Autodesk Inventor part; units mm, degrees
(part 2 of 2)
sketch "Sketch5" plane through (0, 0, 0) normal (0, 0, -1) x (-1, 0, 0)
  arc A0 (-2.4, 16.6775) -> (-3.5193, 18.4731) centre (-4.4, 16.6775) ccw projected
  arc A1 (-3.5193, 28.9932) -> (-3.5193, 18.4731) centre (-0.9394, 23.7332) ccw projected
  arc A2 (-3.5193, 28.9932) -> (-2.4, 30.7889) centre (-4.4, 30.7889) ccw projected
  line L0 (-2.4, 30.7889) -> (-2.4, 61.2014) projected
  arc A3 (-0.4014, 63.2014) -> (-2.4, 61.2014) centre (-0.4, 61.2014) ccw projected
  line L1 (-0.4014, 63.2014) -> (15.0542, 63.2118) projected
  line L2 (15.0542, 63.2118) -> (15, 62.8) projected
  line L3 (15, 62.8) -> (15.1704, 61.5059) projected
  line L4 (15.1704, 61.5059) -> (15.6699, 60.3) projected
  line L5 (15.6699, 60.3) -> (16.4645, 59.2645) projected
  line L6 (16.4645, 59.2645) -> (17.5, 58.4699) projected
  line L7 (17.5, 58.4699) -> (18.7059, 57.9704) projected
  line L8 (18.7059, 57.9704) -> (20, 57.8) projected
  line L9 (20, 57.8) -> (21.2941, 57.9704) projected
  line L10 (21.2941, 57.9704) -> (22.5, 58.4699) projected
  line L11 (22.5, 58.4699) -> (23.5355, 59.2645) projected
  line L12 (23.5355, 59.2645) -> (24.3301, 60.3) projected
  line L13 (24.3301, 60.3) -> (24.8296, 61.5059) projected
  line L14 (24.8296, 61.5059) -> (25, 62.8) projected
  line L15 (25, 62.8) -> (24.9458, 63.212) projected
  line L16 (24.9458, 63.212) -> (130.4002, 63.2002) projected
  arc A4 (132.4, 61.2002) -> (130.4002, 63.2002) centre (130.4, 61.2002) ccw projected
  line L17 (132.4, 61.2002) -> (132.4, 57.5029) projected
  line L18 (132.4, 57.5029) -> (131.5, 57.1301) projected
  line L19 (131.5, 57.1301) -> (130.4645, 56.3355) projected
  line L20 (130.4645, 56.3355) -> (129.6699, 55.3) projected
  line L21 (129.6699, 55.3) -> (129.1704, 54.0941) projected
  line L22 (129.1704, 54.0941) -> (129, 52.8) projected
  line L23 (129, 52.8) -> (129.1704, 51.5059) projected
  line L24 (129.1704, 51.5059) -> (129.6699, 50.3) projected
  line L25 (129.6699, 50.3) -> (130.4645, 49.2645) projected
  line L26 (130.4645, 49.2645) -> (131.5, 48.4699) projected
  line L27 (131.5, 48.4699) -> (132.4, 48.0971) projected
  line L28 (132.4, 48.0971) -> (132.4, -5.0172) projected
  arc A5 (131.3636, -6.7698) -> (132.4, -5.0172) centre (130.4, -5.0172) ccw projected
  line L29 (131.3636, -6.7698) -> (128.4686, -8.3615) projected
  arc A6 (127.505, -8.6089) -> (128.4686, -8.3615) centre (127.505, -6.6089) ccw projected
  line L30 (127.505, -8.6089) -> (2.6647, -8.6089) projected
  arc A7 (1.7321, -8.3782) -> (2.6647, -8.6089) centre (2.6647, -6.6089) ccw projected
  line L31 (1.7321, -8.3782) -> (-1.3326, -6.7626) projected
  arc A8 (-2.4, -4.9934) -> (-1.3326, -6.7626) centre (-0.4, -4.9934) ccw projected
  line L32 (-2.4, -4.9934) -> (-2.4, 16.6775) projected
  line L33 (142.6617, 57.45) -> (142.392, 58.1012) projected
  line L34 (142.392, 58.1012) -> (142.3, 58.8) projected
  line L35 (142.3, 58.8) -> (142.392, 59.4988) projected
  line L36 (142.392, 59.4988) -> (142.6617, 60.15) projected
  line L37 (142.6617, 60.15) -> (143.0908, 60.7092) projected
  line L38 (143.0908, 60.7092) -> (143.65, 61.1383) projected
  line L39 (143.65, 61.1383) -> (144.3012, 61.408) projected
  line L40 (144.3012, 61.408) -> (145, 61.5) projected
  line L41 (145, 61.5) -> (145.6988, 61.408) projected
  line L42 (145.6988, 61.408) -> (146.35, 61.1383) projected
  line L43 (146.35, 61.1383) -> (146.9092, 60.7092) projected
  line L44 (146.9092, 60.7092) -> (147.3383, 60.15) projected
  line L45 (147.3383, 60.15) -> (147.608, 59.4988) projected
  line L46 (147.608, 59.4988) -> (147.7, 58.8) projected
  line L47 (147.7, 58.8) -> (147.608, 58.1012) projected
  line L48 (147.608, 58.1012) -> (147.3383, 57.45) projected
  line L49 (147.3383, 57.45) -> (146.9092, 56.8908) projected
  line L50 (146.9092, 56.8908) -> (146.35, 56.4617) projected
  line L51 (146.35, 56.4617) -> (145.6988, 56.192) projected
  line L52 (145.6988, 56.192) -> (145, 56.1) projected
  line L53 (145, 56.1) -> (144.3012, 56.192) projected
  line L54 (144.3012, 56.192) -> (143.65, 56.4617) projected
  line L55 (143.65, 56.4617) -> (143.0908, 56.8908) projected
  line L56 (143.0908, 56.8908) -> (142.6617, 57.45) projected
  line L57 (-13.0908, -9.2908) -> (-12.6617, -9.85) projected
  line L58 (-12.6617, -9.85) -> (-12.392, -10.5012) projected
  line L59 (-12.392, -10.5012) -> (-12.3, -11.2) projected
  line L60 (-12.3, -11.2) -> (-12.392, -11.8988) projected
  line L61 (-12.392, -11.8988) -> (-12.6617, -12.55) projected
  line L62 (-12.6617, -12.55) -> (-13.0908, -13.1092) projected
  line L63 (-13.0908, -13.1092) -> (-13.65, -13.5383) projected
  line L64 (-13.65, -13.5383) -> (-14.3012, -13.808) projected
  line L65 (-14.3012, -13.808) -> (-15, -13.9) projected
  line L66 (-15, -13.9) -> (-15.6988, -13.808) projected
  line L67 (-15.6988, -13.808) -> (-16.35, -13.5383) projected
  line L68 (-16.35, -13.5383) -> (-16.9092, -13.1092) projected
  line L69 (-16.9092, -13.1092) -> (-17.3383, -12.55) projected
  line L70 (-17.3383, -12.55) -> (-17.608, -11.8988) projected
  line L71 (-17.608, -11.8988) -> (-17.7, -11.2) projected
  line L72 (-17.7, -11.2) -> (-17.608, -10.5012) projected
  line L73 (-17.608, -10.5012) -> (-17.3383, -9.85) projected
  line L74 (-17.3383, -9.85) -> (-16.9092, -9.2908) projected
  line L75 (-16.9092, -9.2908) -> (-16.35, -8.8617) projected
  line L76 (-16.35, -8.8617) -> (-15.6988, -8.592) projected
  line L77 (-15.6988, -8.592) -> (-15, -8.5) projected
  line L78 (-15, -8.5) -> (-14.3012, -8.592) projected
  line L79 (-14.3012, -8.592) -> (-13.65, -8.8617) projected
  line L80 (-13.65, -8.8617) -> (-13.0908, -9.2908) projected
  line L81 (142.6617, -12.55) -> (142.392, -11.8988) projected
  line L82 (142.392, -11.8988) -> (142.3, -11.2) projected
  line L83 (142.3, -11.2) -> (142.392, -10.5012) projected
  line L84 (142.392, -10.5012) -> (142.6617, -9.85) projected
  line L85 (142.6617, -9.85) -> (143.0908, -9.2908) projected
  line L86 (143.0908, -9.2908) -> (143.65, -8.8617) projected
  line L87 (143.65, -8.8617) -> (144.3012, -8.592) projected
  line L88 (144.3012, -8.592) -> (145, -8.5) projected
  line L89 (145, -8.5) -> (145.6988, -8.592) projected
  line L90 (145.6988, -8.592) -> (146.35, -8.8617) projected
  line L91 (146.35, -8.8617) -> (146.9092, -9.2908) projected
  line L92 (146.9092, -9.2908) -> (147.3383, -9.85) projected
  line L93 (147.3383, -9.85) -> (147.608, -10.5012) projected
  line L94 (147.608, -10.5012) -> (147.7, -11.2) projected
  line L95 (147.7, -11.2) -> (147.608, -11.8988) projected
  line L96 (147.608, -11.8988) -> (147.3383, -12.55) projected
  line L97 (147.3383, -12.55) -> (146.9092, -13.1092) projected
  line L98 (146.9092, -13.1092) -> (146.35, -13.5383) projected
  line L99 (146.35, -13.5383) -> (145.6988, -13.808) projected
  line L100 (145.6988, -13.808) -> (145, -13.9) projected
  line L101 (145, -13.9) -> (144.3012, -13.808) projected
  line L102 (144.3012, -13.808) -> (143.65, -13.5383) projected
  line L103 (143.65, -13.5383) -> (143.0908, -13.1092) projected
  line L104 (143.0908, -13.1092) -> (142.6617, -12.55) projected
  line L105 (143.3271, 8.2886) -> (142.7, 8.5483) projected
  line L106 (142.7, 8.5483) -> (142.1615, 8.9615) projected
  line L107 (142.1615, 8.9615) -> (141.7483, 9.5) projected
  line L108 (141.7483, 9.5) -> (141.4886, 10.1271) projected
  line L109 (141.4886, 10.1271) -> (141.4, 10.8) projected
  line L110 (141.4, 10.8) -> (141.4886, 11.4729) projected
  line L111 (141.4886, 11.4729) -> (141.7483, 12.1) projected
  line L112 (141.7483, 12.1) -> (142.1615, 12.6385) projected
  line L113 (142.1615, 12.6385) -> (142.7, 13.0517) projected
  line L114 (142.7, 13.0517) -> (143.3271, 13.3114) projected
  line L115 (143.3271, 13.3114) -> (144, 13.4) projected
  line L116 (144, 13.4) -> (144.6729, 13.3114) projected
  line L117 (144.6729, 13.3114) -> (145.3, 13.0517) projected
  line L118 (145.3, 13.0517) -> (145.8385, 12.6385) projected
  line L119 (145.8385, 12.6385) -> (146.2517, 12.1) projected
  line L120 (146.2517, 12.1) -> (146.5114, 11.4729) projected
  line L121 (146.5114, 11.4729) -> (146.6, 10.8) projected
  line L122 (146.6, 10.8) -> (146.5114, 10.1271) projected
  line L123 (146.5114, 10.1271) -> (146.2517, 9.5) projected
  line L124 (146.2517, 9.5) -> (145.8385, 8.9615) projected
  line L125 (145.8385, 8.9615) -> (145.3, 8.5483) projected
  line L126 (145.3, 8.5483) -> (144.6729, 8.2886) projected
  line L127 (144.6729, 8.2886) -> (144, 8.2) projected
  line L128 (144, 8.2) -> (143.3271, 8.2886) projected
  line L129 (21.8385, 78.9615) -> (21.3, 78.5483) projected
  line L130 (21.3, 78.5483) -> (20.6729, 78.2886) projected
  line L131 (20.6729, 78.2886) -> (20, 78.2) projected
  line L132 (20, 78.2) -> (19.3271, 78.2886) projected
  line L133 (19.3271, 78.2886) -> (18.7, 78.5483) projected
  line L134 (18.7, 78.5483) -> (18.1615, 78.9615) projected
  line L135 (18.1615, 78.9615) -> (17.7483, 79.5) projected
  line L136 (17.7483, 79.5) -> (17.4886, 80.1271) projected
  line L137 (17.4886, 80.1271) -> (17.4, 80.8) projected
  line L138 (17.4, 80.8) -> (17.4886, 81.4729) projected
  line L139 (17.4886, 81.4729) -> (17.7483, 82.1) projected
  line L140 (17.7483, 82.1) -> (18.1615, 82.6385) projected
  line L141 (18.1615, 82.6385) -> (18.7, 83.0517) projected
  line L142 (18.7, 83.0517) -> (19.3271, 83.3114) projected
  line L143 (19.3271, 83.3114) -> (20, 83.4) projected
  line L144 (20, 83.4) -> (20.6729, 83.3114) projected
  line L145 (20.6729, 83.3114) -> (21.3, 83.0517) projected
  line L146 (21.3, 83.0517) -> (21.8385, 82.6385) projected
  line L147 (21.8385, 82.6385) -> (22.2517, 82.1) projected
  line L148 (22.2517, 82.1) -> (22.5114, 81.4729) projected
  line L149 (22.5114, 81.4729) -> (22.6, 80.8) projected
  line L150 (22.6, 80.8) -> (22.5114, 80.1271) projected
  line L151 (22.5114, 80.1271) -> (22.2517, 79.5) projected
  line L152 (22.2517, 79.5) -> (21.8385, 78.9615) projected
  line L153 (110.6729, 78.2886) -> (110, 78.2) projected
  line L154 (110, 78.2) -> (109.3271, 78.2886) projected
  line L155 (109.3271, 78.2886) -> (108.7, 78.5483) projected
  line L156 (108.7, 78.5483) -> (108.1615, 78.9615) projected
  line L157 (108.1615, 78.9615) -> (107.7483, 79.5) projected
  line L158 (107.7483, 79.5) -> (107.4886, 80.1271) projected
  line L159 (107.4886, 80.1271) -> (107.4, 80.8) projected
  line L160 (107.4, 80.8) -> (107.4886, 81.4729) projected
  line L161 (107.4886, 81.4729) -> (107.7483, 82.1) projected
  line L162 (107.7483, 82.1) -> (108.1615, 82.6385) projected
  line L163 (108.1615, 82.6385) -> (108.7, 83.0517) projected
  line L164 (108.7, 83.0517) -> (109.3271, 83.3114) projected
  line L165 (109.3271, 83.3114) -> (110, 83.4) projected
  line L166 (110, 83.4) -> (110.6729, 83.3114) projected
  line L167 (110.6729, 83.3114) -> (111.3, 83.0517) projected
  line L168 (111.3, 83.0517) -> (111.8385, 82.6385) projected
  line L169 (111.8385, 82.6385) -> (112.2517, 82.1) projected
  line L170 (112.2517, 82.1) -> (112.5114, 81.4729) projected
  line L171 (112.5114, 81.4729) -> (112.6, 80.8) projected
  line L172 (112.6, 80.8) -> (112.5114, 80.1271) projected
  line L173 (112.5114, 80.1271) -> (112.2517, 79.5) projected
  line L174 (112.2517, 79.5) -> (111.8385, 78.9615) projected
  line L175 (111.8385, 78.9615) -> (111.3, 78.5483) projected
  line L176 (111.3, 78.5483) -> (110.6729, 78.2886) projected
  line L177 (-12.7, 8.5483) -> (-13.3271, 8.2886) projected
  line L178 (-13.3271, 8.2886) -> (-14, 8.2) projected
  line L179 (-14, 8.2) -> (-14.6729, 8.2886) projected
  line L180 (-14.6729, 8.2886) -> (-15.3, 8.5483) projected
  line L181 (-15.3, 8.5483) -> (-15.8385, 8.9615) projected
  line L182 (-15.8385, 8.9615) -> (-16.2517, 9.5) projected
  line L183 (-16.2517, 9.5) -> (-16.5114, 10.1271) projected
  line L184 (-16.5114, 10.1271) -> (-16.6, 10.8) projected
  line L185 (-16.6, 10.8) -> (-16.5114, 11.4729) projected
  line L186 (-16.5114, 11.4729) -> (-16.2517, 12.1) projected
  line L187 (-16.2517, 12.1) -> (-15.8385, 12.6385) projected
  line L188 (-15.8385, 12.6385) -> (-15.3, 13.0517) projected
  line L189 (-15.3, 13.0517) -> (-14.6729, 13.3114) projected
  line L190 (-14.6729, 13.3114) -> (-14, 13.4) projected
  line L191 (-14, 13.4) -> (-13.3271, 13.3114) projected
  line L192 (-13.3271, 13.3114) -> (-12.7, 13.0517) projected
  line L193 (-12.7, 13.0517) -> (-12.1615, 12.6385) projected
  line L194 (-12.1615, 12.6385) -> (-11.7483, 12.1) projected
  line L195 (-11.7483, 12.1) -> (-11.4886, 11.4729) projected
  line L196 (-11.4886, 11.4729) -> (-11.4, 10.8) projected
  line L197 (-11.4, 10.8) -> (-11.4886, 10.1271) projected
  line L198 (-11.4886, 10.1271) -> (-11.7483, 9.5) projected
  line L199 (-11.7483, 9.5) -> (-12.1615, 8.9615) projected
  line L200 (-12.1615, 8.9615) -> (-12.7, 8.5483) projected
  line L201 (147.8159, -4.2) -> (147.8159, -7.2) projected
  line L202 (147.8159, -7.2) -> (142.8159, -7.2) projected
  line L203 (142.8159, -7.2) -> (142.8159, -4.2) projected
  line L204 (142.8159, -4.2) -> (147.8159, -4.2) projected
  line L205 (133.2, 51.4144) -> (132.8686, 51.6686) projected
  line L206 (132.8686, 51.6686) -> (132.6144, 52) projected
  line L207 (132.6144, 52) -> (132.4545, 52.3859) projected
  line L208 (132.4545, 52.3859) -> (132.4, 52.8) projected
  line L209 (132.4, 52.8) -> (132.4545, 53.2141) projected
  line L210 (132.4545, 53.2141) -> (132.6144, 53.6) projected
  line L211 (132.6144, 53.6) -> (132.8686, 53.9314) projected
  line L212 (132.8686, 53.9314) -> (133.2, 54.1856) projected
  line L213 (133.2, 54.1856) -> (133.5859, 54.3455) projected
  line L214 (133.5859, 54.3455) -> (134, 54.4) projected
  line L215 (134, 54.4) -> (134.4141, 54.3455) projected
  line L216 (134.4141, 54.3455) -> (134.8, 54.1856) projected
  line L217 (134.8, 54.1856) -> (135.1314, 53.9314) projected
  line L218 (135.1314, 53.9314) -> (135.3856, 53.6) projected
  line L219 (135.3856, 53.6) -> (135.5455, 53.2141) projected
  line L220 (135.5455, 53.2141) -> (135.6, 52.8) projected
  line L221 (135.6, 52.8) -> (135.5455, 52.3859) projected
  line L222 (135.5455, 52.3859) -> (135.3856, 52) projected
  line L223 (135.3856, 52) -> (135.1314, 51.6686) projected
  line L224 (135.1314, 51.6686) -> (134.8, 51.4144) projected
  line L225 (134.8, 51.4144) -> (134.4141, 51.2545) projected
  line L226 (134.4141, 51.2545) -> (134, 51.2) projected
  line L227 (134, 51.2) -> (133.5859, 51.2545) projected
  line L228 (133.5859, 51.2545) -> (133.2, 51.4144) projected
  line L229 (20, 61.2) -> (19.5859, 61.2545) projected
  line L230 (19.5859, 61.2545) -> (19.2, 61.4144) projected
  line L231 (19.2, 61.4144) -> (18.8686, 61.6686) projected
  line L232 (18.8686, 61.6686) -> (18.6144, 62) projected
  line L233 (18.6144, 62) -> (18.4545, 62.3859) projected
  line L234 (18.4545, 62.3859) -> (18.4, 62.8) projected
  line L235 (18.4, 62.8) -> (18.4545, 63.2141) projected
  line L236 (18.4545, 63.2141) -> (18.6144, 63.6) projected
  line L237 (18.6144, 63.6) -> (18.8686, 63.9314) projected
  line L238 (18.8686, 63.9314) -> (19.2, 64.1856) projected
  line L239 (19.2, 64.1856) -> (19.5859, 64.3455) projected
  line L240 (19.5859, 64.3455) -> (20, 64.4) projected
  line L241 (20, 64.4) -> (20.4141, 64.3455) projected
  line L242 (20.4141, 64.3455) -> (20.8, 64.1856) projected
  line L243 (20.8, 64.1856) -> (21.1314, 63.9314) projected
  line L244 (21.1314, 63.9314) -> (21.3856, 63.6) projected
  line L245 (21.3856, 63.6) -> (21.5455, 63.2141) projected
  line L246 (21.5455, 63.2141) -> (21.6, 62.8) projected
  line L247 (21.6, 62.8) -> (21.5455, 62.3859) projected
  line L248 (21.5455, 62.3859) -> (21.3856, 62) projected
  line L249 (21.3856, 62) -> (21.1314, 61.6686) projected
  line L250 (21.1314, 61.6686) -> (20.8, 61.4144) projected
  line L251 (20.8, 61.4144) -> (20.4141, 61.2545) projected
  line L252 (20.4141, 61.2545) -> (20, 61.2) projected
  line L253 (-5.1314, -12.3314) -> (-5.3856, -12) projected
  line L254 (-5.3856, -12) -> (-5.5455, -11.6141) projected
  line L255 (-5.5455, -11.6141) -> (-5.6, -11.2) projected
  line L256 (-5.6, -11.2) -> (-5.5455, -10.7859) projected
  line L257 (-5.5455, -10.7859) -> (-5.3856, -10.4) projected
  line L258 (-5.3856, -10.4) -> (-5.1314, -10.0686) projected
  line L259 (-5.1314, -10.0686) -> (-4.8, -9.8144) projected
  line L260 (-4.8, -9.8144) -> (-4.4141, -9.6545) projected
  line L261 (-4.4141, -9.6545) -> (-4, -9.6) projected
  line L262 (-4, -9.6) -> (-3.5859, -9.6545) projected
  line L263 (-3.5859, -9.6545) -> (-3.2, -9.8144) projected
  line L264 (-3.2, -9.8144) -> (-2.8686, -10.0686) projected
  line L265 (-2.8686, -10.0686) -> (-2.6144, -10.4) projected
  line L266 (-2.6144, -10.4) -> (-2.4545, -10.7859) projected
  line L267 (-2.4545, -10.7859) -> (-2.4, -11.2) projected
  line L268 (-2.4, -11.2) -> (-2.4545, -11.6141) projected
  line L269 (-2.4545, -11.6141) -> (-2.6144, -12) projected
  line L270 (-2.6144, -12) -> (-2.8686, -12.3314) projected
  line L271 (-2.8686, -12.3314) -> (-3.2, -12.5856) projected
  line L272 (-3.2, -12.5856) -> (-3.5859, -12.7455) projected
  line L273 (-3.5859, -12.7455) -> (-4, -12.8) projected
  line L274 (-4, -12.8) -> (-4.4141, -12.7455) projected
  line L275 (-4.4141, -12.7455) -> (-4.8, -12.5856) projected
  line L276 (-4.8, -12.5856) -> (-5.1314, -12.3314) projected
  line L277 (135.3856, -10.4) -> (135.5455, -10.7859) projected
  line L278 (135.5455, -10.7859) -> (135.6, -11.2) projected
  line L279 (135.6, -11.2) -> (135.5455, -11.6141) projected
  line L280 (135.5455, -11.6141) -> (135.3856, -12) projected
  line L281 (135.3856, -12) -> (135.1314, -12.3314) projected
  line L282 (135.1314, -12.3314) -> (134.8, -12.5856) projected
  line L283 (134.8, -12.5856) -> (134.4141, -12.7455) projected
  line L284 (134.4141, -12.7455) -> (134, -12.8) projected
  line L285 (134, -12.8) -> (133.5859, -12.7455) projected
  line L286 (133.5859, -12.7455) -> (133.2, -12.5856) projected
  line L287 (133.2, -12.5856) -> (132.8686, -12.3314) projected
  line L288 (132.8686, -12.3314) -> (132.6144, -12) projected
  line L289 (132.6144, -12) -> (132.4545, -11.6141) projected
  line L290 (132.4545, -11.6141) -> (132.4, -11.2) projected
  line L291 (132.4, -11.2) -> (132.4545, -10.7859) projected
  line L292 (132.4545, -10.7859) -> (132.6144, -10.4) projected
  line L293 (132.6144, -10.4) -> (132.8686, -10.0686) projected
  line L294 (132.8686, -10.0686) -> (133.2, -9.8144) projected
  line L295 (133.2, -9.8144) -> (133.5859, -9.6545) projected
  line L296 (133.5859, -9.6545) -> (134, -9.6) projected
  line L297 (134, -9.6) -> (134.4141, -9.6545) projected
  line L298 (134.4141, -9.6545) -> (134.8, -9.8144) projected
  line L299 (134.8, -9.8144) -> (135.1314, -10.0686) projected
  line L300 (135.1314, -10.0686) -> (135.3856, -10.4) projected
  line L301 (-18, 19.2664) -> (-13, 19.2664) projected
  arc A9 (-18, 19.2664) -> (-20, 17.2664) centre (-18, 17.2664) ccw projected
  line L302 (-20, -15.2) -> (-20, 17.2664) projected
  line L303 (-19.9319, -15.7176) -> (-20, -15.2) projected
  line L304 (-19.8478, -15.9654) -> (-19.9319, -15.7176) projected
  line L305 (-19.7321, -16.2) -> (-19.8478, -15.9654) projected
  line L306 (-19.5867, -16.4175) -> (-19.7321, -16.2) projected
  line L307 (-19.4142, -16.6142) -> (-19.5867, -16.4175) projected
  line L308 (-19.2175, -16.7867) -> (-19.4142, -16.6142) projected
  line L309 (-19, -16.9321) -> (-19.2175, -16.7867) projected
  line L310 (-18.7654, -17.0478) -> (-19, -16.9321) projected
  line L311 (-18.5176, -17.1319) -> (-18.7654, -17.0478) projected
  line L312 (-18, -17.2) -> (-18.5176, -17.1319) projected
  line L313 (148, -17.2) -> (-18, -17.2) projected
  line L314 (148.5176, -17.1319) -> (148, -17.2) projected
  line L315 (148.7654, -17.0478) -> (148.5176, -17.1319) projected
  line L316 (149, -16.9321) -> (148.7654, -17.0478) projected
  line L317 (149.2175, -16.7867) -> (149, -16.9321) projected
  line L318 (149.4142, -16.6142) -> (149.2175, -16.7867) projected
  line L319 (149.5867, -16.4175) -> (149.4142, -16.6142) projected
  line L320 (149.7321, -16.2) -> (149.5867, -16.4175) projected
  line L321 (149.8478, -15.9654) -> (149.7321, -16.2) projected
  line L322 (149.9319, -15.7176) -> (149.8478, -15.9654) projected
  line L323 (150, -15.2) -> (149.9319, -15.7176) projected
  line L324 (150, 86.8) -> (150, -15.2) projected
  line L325 (149.9319, 87.3176) -> (150, 86.8) projected
  line L326 (149.8478, 87.5654) -> (149.9319, 87.3176) projected
  line L327 (149.7321, 87.8) -> (149.8478, 87.5654) projected
  line L328 (149.5867, 88.0175) -> (149.7321, 87.8) projected
  line L329 (149.4142, 88.2142) -> (149.5867, 88.0175) projected
  line L330 (149.2175, 88.3867) -> (149.4142, 88.2142) projected
  line L331 (149, 88.5321) -> (149.2175, 88.3867) projected
  line L332 (148.7654, 88.6478) -> (149, 88.5321) projected
  line L333 (148.5176, 88.7319) -> (148.7654, 88.6478) projected
  line L334 (148, 88.8) -> (148.5176, 88.7319) projected
  line L335 (-9, 88.8) -> (148, 88.8) projected
  arc A10 (-9, 88.8) -> (-11, 86.8) centre (-9, 86.8) ccw projected
  line L336 (-11, 21.2664) -> (-11, 86.8) projected
  arc A11 (-13, 19.2664) -> (-11, 21.2664) centre (-13, 21.2664) ccw projected
  circle A12 centre (134, -11.2) radius 1.5863
  circle A13 centre (134, 52.8) radius 1.5863
  circle A14 centre (20, 62.8) radius 1.5863
  circle A15 centre (-4, -11.2) radius 1.5863
  point P0 (0, 0)
  constraints: 12 tangent, 4 centre point
hole "Hole1" at (-134, 52.8, 0) at (-134, -11.2, 0) at (-20, 62.8, 0) at (4, -11.2, 0) direction (0, 0, 1) diameter 3.3 end through all
sketch "Sketch6" plane through (0, 0, 0) normal (0, 0, -1) x (-1, 0, 0)
  circle A0 centre (20, 62.8) radius 1.65 projected
  circle A1 centre (134, 52.8) radius 1.65 projected
  circle A2 centre (134, -11.2) radius 1.65 projected
  circle A3 centre (-4, -11.2) radius 1.65 projected
  arc A4 (-2.4, 16.6775) -> (-3.5193, 18.4731) centre (-4.4, 16.6775) ccw projected
  arc A5 (-3.5193, 28.9932) -> (-3.5193, 18.4731) centre (-0.9394, 23.7332) ccw projected
  arc A6 (-3.5193, 28.9932) -> (-2.4, 30.7889) centre (-4.4, 30.7889) ccw projected
  line L0 (-2.4, 30.7889) -> (-2.4, 61.2014) projected
  arc A7 (-0.4014, 63.2014) -> (-2.4, 61.2014) centre (-0.4, 61.2014) ccw projected
  line L1 (-0.4014, 63.2014) -> (15.0542, 63.2118) projected
  line L2 (15.0542, 63.2118) -> (15, 62.8) projected
  line L3 (15, 62.8) -> (15.1704, 61.5059) projected
  line L4 (15.1704, 61.5059) -> (15.6699, 60.3) projected
  line L5 (15.6699, 60.3) -> (16.4645, 59.2645) projected
  line L6 (16.4645, 59.2645) -> (17.5, 58.4699) projected
  line L7 (17.5, 58.4699) -> (18.7059, 57.9704) projected
  line L8 (18.7059, 57.9704) -> (20, 57.8) projected
  line L9 (20, 57.8) -> (21.2941, 57.9704) projected
  line L10 (21.2941, 57.9704) -> (22.5, 58.4699) projected
  line L11 (22.5, 58.4699) -> (23.5355, 59.2645) projected
  line L12 (23.5355, 59.2645) -> (24.3301, 60.3) projected
  line L13 (24.3301, 60.3) -> (24.8296, 61.5059) projected
  line L14 (24.8296, 61.5059) -> (25, 62.8) projected
  line L15 (25, 62.8) -> (24.9458, 63.212) projected
  line L16 (24.9458, 63.212) -> (130.4002, 63.2002) projected
  arc A8 (132.4, 61.2002) -> (130.4002, 63.2002) centre (130.4, 61.2002) ccw projected
  line L17 (132.4, 61.2002) -> (132.4, 57.5029) projected
  line L18 (132.4, 57.5029) -> (131.5, 57.1301) projected
  line L19 (131.5, 57.1301) -> (130.4645, 56.3355) projected
  line L20 (130.4645, 56.3355) -> (129.6699, 55.3) projected
  line L21 (129.6699, 55.3) -> (129.1704, 54.0941) projected
  line L22 (129.1704, 54.0941) -> (129, 52.8) projected
  line L23 (129, 52.8) -> (129.1704, 51.5059) projected
  line L24 (129.1704, 51.5059) -> (129.6699, 50.3) projected
  line L25 (129.6699, 50.3) -> (130.4645, 49.2645) projected
  line L26 (130.4645, 49.2645) -> (131.5, 48.4699) projected
  line L27 (131.5, 48.4699) -> (132.4, 48.0971) projected
  line L28 (132.4, 48.0971) -> (132.4, -5.0172) projected
  arc A9 (131.3636, -6.7698) -> (132.4, -5.0172) centre (130.4, -5.0172) ccw projected
  line L29 (131.3636, -6.7698) -> (128.4686, -8.3615) projected
  arc A10 (127.505, -8.6089) -> (128.4686, -8.3615) centre (127.505, -6.6089) ccw projected
  line L30 (127.505, -8.6089) -> (2.6647, -8.6089) projected
  arc A11 (1.7321, -8.3782) -> (2.6647, -8.6089) centre (2.6647, -6.6089) ccw projected
  line L31 (1.7321, -8.3782) -> (-1.3326, -6.7626) projected
  arc A12 (-2.4, -4.9934) -> (-1.3326, -6.7626) centre (-0.4, -4.9934) ccw projected
  line L32 (-2.4, -4.9934) -> (-2.4, 16.6775) projected
  line L33 (142.6617, 57.45) -> (142.392, 58.1012) projected
  line L34 (142.392, 58.1012) -> (142.3, 58.8) projected
  line L35 (142.3, 58.8) -> (142.392, 59.4988) projected
  line L36 (142.392, 59.4988) -> (142.6617, 60.15) projected
  line L37 (142.6617, 60.15) -> (143.0908, 60.7092) projected
  line L38 (143.0908, 60.7092) -> (143.65, 61.1383) projected
  line L39 (143.65, 61.1383) -> (144.3012, 61.408) projected
  line L40 (144.3012, 61.408) -> (145, 61.5) projected
  line L41 (145, 61.5) -> (145.6988, 61.408) projected
  line L42 (145.6988, 61.408) -> (146.35, 61.1383) projected
  line L43 (146.35, 61.1383) -> (146.9092, 60.7092) projected
  line L44 (146.9092, 60.7092) -> (147.3383, 60.15) projected
  line L45 (147.3383, 60.15) -> (147.608, 59.4988) projected
  line L46 (147.608, 59.4988) -> (147.7, 58.8) projected
  line L47 (147.7, 58.8) -> (147.608, 58.1012) projected
  line L48 (147.608, 58.1012) -> (147.3383, 57.45) projected
  line L49 (147.3383, 57.45) -> (146.9092, 56.8908) projected
  line L50 (146.9092, 56.8908) -> (146.35, 56.4617) projected
  line L51 (146.35, 56.4617) -> (145.6988, 56.192) projected
  line L52 (145.6988, 56.192) -> (145, 56.1) projected
  line L53 (145, 56.1) -> (144.3012, 56.192) projected
  line L54 (144.3012, 56.192) -> (143.65, 56.4617) projected
  line L55 (143.65, 56.4617) -> (143.0908, 56.8908) projected
  line L56 (143.0908, 56.8908) -> (142.6617, 57.45) projected
  line L57 (-13.0908, -9.2908) -> (-12.6617, -9.85) projected
  line L58 (-12.6617, -9.85) -> (-12.392, -10.5012) projected
  line L59 (-12.392, -10.5012) -> (-12.3, -11.2) projected
  line L60 (-12.3, -11.2) -> (-12.392, -11.8988) projected
  line L61 (-12.392, -11.8988) -> (-12.6617, -12.55) projected
  line L62 (-12.6617, -12.55) -> (-13.0908, -13.1092) projected
  line L63 (-13.0908, -13.1092) -> (-13.65, -13.5383) projected
  line L64 (-13.65, -13.5383) -> (-14.3012, -13.808) projected
  line L65 (-14.3012, -13.808) -> (-15, -13.9) projected
  line L66 (-15, -13.9) -> (-15.6988, -13.808) projected
  line L67 (-15.6988, -13.808) -> (-16.35, -13.5383) projected
  line L68 (-16.35, -13.5383) -> (-16.9092, -13.1092) projected
  line L69 (-16.9092, -13.1092) -> (-17.3383, -12.55) projected
  line L70 (-17.3383, -12.55) -> (-17.608, -11.8988) projected
  line L71 (-17.608, -11.8988) -> (-17.7, -11.2) projected
  line L72 (-17.7, -11.2) -> (-17.608, -10.5012) projected
  line L73 (-17.608, -10.5012) -> (-17.3383, -9.85) projected
  line L74 (-17.3383, -9.85) -> (-16.9092, -9.2908) projected
  line L75 (-16.9092, -9.2908) -> (-16.35, -8.8617) projected
  line L76 (-16.35, -8.8617) -> (-15.6988, -8.592) projected
  line L77 (-15.6988, -8.592) -> (-15, -8.5) projected
  line L78 (-15, -8.5) -> (-14.3012, -8.592) projected
  line L79 (-14.3012, -8.592) -> (-13.65, -8.8617) projected
  line L80 (-13.65, -8.8617) -> (-13.0908, -9.2908) projected
  line L81 (142.6617, -12.55) -> (142.392, -11.8988) projected
  line L82 (142.392, -11.8988) -> (142.3, -11.2) projected
  line L83 (142.3, -11.2) -> (142.392, -10.5012) projected
  line L84 (142.392, -10.5012) -> (142.6617, -9.85) projected
  line L85 (142.6617, -9.85) -> (143.0908, -9.2908) projected
  line L86 (143.0908, -9.2908) -> (143.65, -8.8617) projected
  line L87 (143.65, -8.8617) -> (144.3012, -8.592) projected
  line L88 (144.3012, -8.592) -> (145, -8.5) projected
  line L89 (145, -8.5) -> (145.6988, -8.592) projected
  line L90 (145.6988, -8.592) -> (146.35, -8.8617) projected
  line L91 (146.35, -8.8617) -> (146.9092, -9.2908) projected
  line L92 (146.9092, -9.2908) -> (147.3383, -9.85) projected
  line L93 (147.3383, -9.85) -> (147.608, -10.5012) projected
  line L94 (147.608, -10.5012) -> (147.7, -11.2) projected
  line L95 (147.7, -11.2) -> (147.608, -11.8988) projected
  line L96 (147.608, -11.8988) -> (147.3383, -12.55) projected
  line L97 (147.3383, -12.55) -> (146.9092, -13.1092) projected
  line L98 (146.9092, -13.1092) -> (146.35, -13.5383) projected
  line L99 (146.35, -13.5383) -> (145.6988, -13.808) projected
  line L100 (145.6988, -13.808) -> (145, -13.9) projected
  line L101 (145, -13.9) -> (144.3012, -13.808) projected
  line L102 (144.3012, -13.808) -> (143.65, -13.5383) projected
  line L103 (143.65, -13.5383) -> (143.0908, -13.1092) projected
  line L104 (143.0908, -13.1092) -> (142.6617, -12.55) projected
  line L105 (143.3271, 8.2886) -> (142.7, 8.5483) projected
  line L106 (142.7, 8.5483) -> (142.1615, 8.9615) projected
  line L107 (142.1615, 8.9615) -> (141.7483, 9.5) projected
  line L108 (141.7483, 9.5) -> (141.4886, 10.1271) projected
  line L109 (141.4886, 10.1271) -> (141.4, 10.8) projected
  line L110 (141.4, 10.8) -> (141.4886, 11.4729) projected
  line L111 (141.4886, 11.4729) -> (141.7483, 12.1) projected
  line L112 (141.7483, 12.1) -> (142.1615, 12.6385) projected
  line L113 (142.1615, 12.6385) -> (142.7, 13.0517) projected
  line L114 (142.7, 13.0517) -> (143.3271, 13.3114) projected
  line L115 (143.3271, 13.3114) -> (144, 13.4) projected
  line L116 (144, 13.4) -> (144.6729, 13.3114) projected
  line L117 (144.6729, 13.3114) -> (145.3, 13.0517) projected
  line L118 (145.3, 13.0517) -> (145.8385, 12.6385) projected
  line L119 (145.8385, 12.6385) -> (146.2517, 12.1) projected
  line L120 (146.2517, 12.1) -> (146.5114, 11.4729) projected
  line L121 (146.5114, 11.4729) -> (146.6, 10.8) projected
  line L122 (146.6, 10.8) -> (146.5114, 10.1271) projected
  line L123 (146.5114, 10.1271) -> (146.2517, 9.5) projected
  line L124 (146.2517, 9.5) -> (145.8385, 8.9615) projected
  line L125 (145.8385, 8.9615) -> (145.3, 8.5483) projected
  line L126 (145.3, 8.5483) -> (144.6729, 8.2886) projected
  line L127 (144.6729, 8.2886) -> (144, 8.2) projected
  line L128 (144, 8.2) -> (143.3271, 8.2886) projected
  line L129 (21.8385, 78.9615) -> (21.3, 78.5483) projected
  line L130 (21.3, 78.5483) -> (20.6729, 78.2886) projected
  line L131 (20.6729, 78.2886) -> (20, 78.2) projected
  line L132 (20, 78.2) -> (19.3271, 78.2886) projected
  line L133 (19.3271, 78.2886) -> (18.7, 78.5483) projected
  line L134 (18.7, 78.5483) -> (18.1615, 78.9615) projected
  line L135 (18.1615, 78.9615) -> (17.7483, 79.5) projected
  line L136 (17.7483, 79.5) -> (17.4886, 80.1271) projected
  line L137 (17.4886, 80.1271) -> (17.4, 80.8) projected
  line L138 (17.4, 80.8) -> (17.4886, 81.4729) projected
  line L139 (17.4886, 81.4729) -> (17.7483, 82.1) projected
  line L140 (17.7483, 82.1) -> (18.1615, 82.6385) projected
  line L141 (18.1615, 82.6385) -> (18.7, 83.0517) projected
  line L142 (18.7, 83.0517) -> (19.3271, 83.3114) projected
  line L143 (19.3271, 83.3114) -> (20, 83.4) projected
  line L144 (20, 83.4) -> (20.6729, 83.3114) projected
  line L145 (20.6729, 83.3114) -> (21.3, 83.0517) projected
  line L146 (21.3, 83.0517) -> (21.8385, 82.6385) projected
  line L147 (21.8385, 82.6385) -> (22.2517, 82.1) projected
  line L148 (22.2517, 82.1) -> (22.5114, 81.4729) projected
  line L149 (22.5114, 81.4729) -> (22.6, 80.8) projected
  line L150 (22.6, 80.8) -> (22.5114, 80.1271) projected
  line L151 (22.5114, 80.1271) -> (22.2517, 79.5) projected
  line L152 (22.2517, 79.5) -> (21.8385, 78.9615) projected
  line L153 (110.6729, 78.2886) -> (110, 78.2) projected
  line L154 (110, 78.2) -> (109.3271, 78.2886) projected
  line L155 (109.3271, 78.2886) -> (108.7, 78.5483) projected
  line L156 (108.7, 78.5483) -> (108.1615, 78.9615) projected
  line L157 (108.1615, 78.9615) -> (107.7483, 79.5) projected
  line L158 (107.7483, 79.5) -> (107.4886, 80.1271) projected
  line L159 (107.4886, 80.1271) -> (107.4, 80.8) projected
  line L160 (107.4, 80.8) -> (107.4886, 81.4729) projected
  line L161 (107.4886, 81.4729) -> (107.7483, 82.1) projected
  line L162 (107.7483, 82.1) -> (108.1615, 82.6385) projected
  line L163 (108.1615, 82.6385) -> (108.7, 83.0517) projected
  line L164 (108.7, 83.0517) -> (109.3271, 83.3114) projected
  line L165 (109.3271, 83.3114) -> (110, 83.4) projected
  line L166 (110, 83.4) -> (110.6729, 83.3114) projected
  line L167 (110.6729, 83.3114) -> (111.3, 83.0517) projected
  line L168 (111.3, 83.0517) -> (111.8385, 82.6385) projected
  line L169 (111.8385, 82.6385) -> (112.2517, 82.1) projected
  line L170 (112.2517, 82.1) -> (112.5114, 81.4729) projected
  line L171 (112.5114, 81.4729) -> (112.6, 80.8) projected
  line L172 (112.6, 80.8) -> (112.5114, 80.1271) projected
  line L173 (112.5114, 80.1271) -> (112.2517, 79.5) projected
  line L174 (112.2517, 79.5) -> (111.8385, 78.9615) projected
  line L175 (111.8385, 78.9615) -> (111.3, 78.5483) projected
  line L176 (111.3, 78.5483) -> (110.6729, 78.2886) projected
  line L177 (-12.7, 8.5483) -> (-13.3271, 8.2886) projected
  line L178 (-13.3271, 8.2886) -> (-14, 8.2) projected
  line L179 (-14, 8.2) -> (-14.6729, 8.2886) projected
  line L180 (-14.6729, 8.2886) -> (-15.3, 8.5483) projected
  line L181 (-15.3, 8.5483) -> (-15.8385, 8.9615) projected
  line L182 (-15.8385, 8.9615) -> (-16.2517, 9.5) projected
  line L183 (-16.2517, 9.5) -> (-16.5114, 10.1271) projected
  line L184 (-16.5114, 10.1271) -> (-16.6, 10.8) projected
  line L185 (-16.6, 10.8) -> (-16.5114, 11.4729) projected
  line L186 (-16.5114, 11.4729) -> (-16.2517, 12.1) projected
  line L187 (-16.2517, 12.1) -> (-15.8385, 12.6385) projected
  line L188 (-15.8385, 12.6385) -> (-15.3, 13.0517) projected
  line L189 (-15.3, 13.0517) -> (-14.6729, 13.3114) projected
  line L190 (-14.6729, 13.3114) -> (-14, 13.4) projected
  line L191 (-14, 13.4) -> (-13.3271, 13.3114) projected
  line L192 (-13.3271, 13.3114) -> (-12.7, 13.0517) projected
  line L193 (-12.7, 13.0517) -> (-12.1615, 12.6385) projected
  line L194 (-12.1615, 12.6385) -> (-11.7483, 12.1) projected
  line L195 (-11.7483, 12.1) -> (-11.4886, 11.4729) projected
  line L196 (-11.4886, 11.4729) -> (-11.4, 10.8) projected
  line L197 (-11.4, 10.8) -> (-11.4886, 10.1271) projected
  line L198 (-11.4886, 10.1271) -> (-11.7483, 9.5) projected
  line L199 (-11.7483, 9.5) -> (-12.1615, 8.9615) projected
  line L200 (-12.1615, 8.9615) -> (-12.7, 8.5483) projected
  line L201 (147.8159, -4.2) -> (147.8159, -7.2) projected
  line L202 (147.8159, -7.2) -> (142.8159, -7.2) projected
  line L203 (142.8159, -7.2) -> (142.8159, -4.2) projected
  line L204 (142.8159, -4.2) -> (147.8159, -4.2) projected
  line L205 (-18, 19.2664) -> (-13, 19.2664) projected
  arc A13 (-18, 19.2664) -> (-20, 17.2664) centre (-18, 17.2664) ccw projected
  line L206 (-20, -15.2) -> (-20, 17.2664) projected
  line L207 (-19.9319, -15.7176) -> (-20, -15.2) projected
  line L208 (-19.8478, -15.9654) -> (-19.9319, -15.7176) projected
  line L209 (-19.7321, -16.2) -> (-19.8478, -15.9654) projected
  line L210 (-19.5867, -16.4175) -> (-19.7321, -16.2) projected
  line L211 (-19.4142, -16.6142) -> (-19.5867, -16.4175) projected
  line L212 (-19.2175, -16.7867) -> (-19.4142, -16.6142) projected
  line L213 (-19, -16.9321) -> (-19.2175, -16.7867) projected
  line L214 (-18.7654, -17.0478) -> (-19, -16.9321) projected
  line L215 (-18.5176, -17.1319) -> (-18.7654, -17.0478) projected
  line L216 (-18, -17.2) -> (-18.5176, -17.1319) projected
  line L217 (148, -17.2) -> (-18, -17.2) projected
  line L218 (148.5176, -17.1319) -> (148, -17.2) projected
  line L219 (148.7654, -17.0478) -> (148.5176, -17.1319) projected
  line L220 (149, -16.9321) -> (148.7654, -17.0478) projected
  line L221 (149.2175, -16.7867) -> (149, -16.9321) projected
  line L222 (149.4142, -16.6142) -> (149.2175, -16.7867) projected
  line L223 (149.5867, -16.4175) -> (149.4142, -16.6142) projected
  line L224 (149.7321, -16.2) -> (149.5867, -16.4175) projected
  line L225 (149.8478, -15.9654) -> (149.7321, -16.2) projected
  line L226 (149.9319, -15.7176) -> (149.8478, -15.9654) projected
  line L227 (150, -15.2) -> (149.9319, -15.7176) projected
  line L228 (150, 86.8) -> (150, -15.2) projected
  line L229 (149.9319, 87.3176) -> (150, 86.8) projected
  line L230 (149.8478, 87.5654) -> (149.9319, 87.3176) projected
  line L231 (149.7321, 87.8) -> (149.8478, 87.5654) projected
  line L232 (149.5867, 88.0175) -> (149.7321, 87.8) projected
  line L233 (149.4142, 88.2142) -> (149.5867, 88.0175) projected
  line L234 (149.2175, 88.3867) -> (149.4142, 88.2142) projected
  line L235 (149, 88.5321) -> (149.2175, 88.3867) projected
  line L236 (148.7654, 88.6478) -> (149, 88.5321) projected
  line L237 (148.5176, 88.7319) -> (148.7654, 88.6478) projected
  line L238 (148, 88.8) -> (148.5176, 88.7319) projected
  line L239 (-9, 88.8) -> (148, 88.8) projected
  arc A14 (-9, 88.8) -> (-11, 86.8) centre (-9, 86.8) ccw projected
  line L240 (-11, 21.2664) -> (-11, 86.8) projected
  arc A15 (-13, 19.2664) -> (-11, 21.2664) centre (-13, 21.2664) ccw projected
  circle A16 centre (145, -11.2) radius 2.6769
  circle A17 centre (144, 10.8) radius 2.5778
  circle A18 centre (145, 58.8) radius 2.6769
  circle A19 centre (110, 80.8) radius 2.5778
  circle A20 centre (20, 80.8) radius 2.5778
  circle A21 centre (-14, 10.8) radius 2.5778
  circle A22 centre (-15, -11.2) radius 2.6769
  point P0 (0, 0)
  constraints: 21 tangent, 7 centre point
hole "Hole2" at (-145, -11.2, 0) at (-144, 10.8, 0) at (15, -11.2, 0) at (14, 10.8, 0) at (-20, 80.8, 0) at (-110, 80.8, 0) at (-145, 58.8, 0) direction (0, 0, 1) diameter 5.4 end through all
sketch "Sketch7" plane through (0, 0, 0) normal (0, 0, -1) x (-1, 0, 0)
  circle A0 centre (145, -11.2) radius 2.7 projected
  circle A1 centre (-15, -11.2) radius 2.7 projected
  circle A2 centre (145, 58.8) radius 2.7 projected
  circle A3 centre (110, 80.8) radius 2.7 projected
  circle A4 centre (-14, 10.8) radius 2.7 projected
  circle A5 centre (144, 10.8) radius 2.7 projected
  circle A6 centre (20, 80.8) radius 2.7 projected
  circle A7 centre (20, 62.8) radius 1.65 projected
  circle A8 centre (134, 52.8) radius 1.65 projected
  circle A9 centre (134, -11.2) radius 1.65 projected
  circle A10 centre (-4, -11.2) radius 1.65 projected
  arc A11 (-2.4, 16.6775) -> (-3.5193, 18.4731) centre (-4.4, 16.6775) ccw projected
  arc A12 (-3.5193, 28.9932) -> (-3.5193, 18.4731) centre (-0.9394, 23.7332) ccw projected
  arc A13 (-3.5193, 28.9932) -> (-2.4, 30.7889) centre (-4.4, 30.7889) ccw projected
  line L0 (-2.4, 30.7889) -> (-2.4, 61.2014) projected
  arc A14 (-0.4014, 63.2014) -> (-2.4, 61.2014) centre (-0.4, 61.2014) ccw projected
  line L1 (-0.4014, 63.2014) -> (15.0542, 63.2118) projected
  line L2 (15.0542, 63.2118) -> (15, 62.8) projected
  line L3 (15, 62.8) -> (15.1704, 61.5059) projected
  line L4 (15.1704, 61.5059) -> (15.6699, 60.3) projected
  line L5 (15.6699, 60.3) -> (16.4645, 59.2645) projected
  line L6 (16.4645, 59.2645) -> (17.5, 58.4699) projected
  line L7 (17.5, 58.4699) -> (18.7059, 57.9704) projected
  line L8 (18.7059, 57.9704) -> (20, 57.8) projected
  line L9 (20, 57.8) -> (21.2941, 57.9704) projected
  line L10 (21.2941, 57.9704) -> (22.5, 58.4699) projected
  line L11 (22.5, 58.4699) -> (23.5355, 59.2645) projected
  line L12 (23.5355, 59.2645) -> (24.3301, 60.3) projected
  line L13 (24.3301, 60.3) -> (24.8296, 61.5059) projected
  line L14 (24.8296, 61.5059) -> (25, 62.8) projected
  line L15 (25, 62.8) -> (24.9458, 63.212) projected
  line L16 (24.9458, 63.212) -> (130.4002, 63.2002) projected
  arc A15 (132.4, 61.2002) -> (130.4002, 63.2002) centre (130.4, 61.2002) ccw projected
  line L17 (132.4, 61.2002) -> (132.4, 57.5029) projected
  line L18 (132.4, 57.5029) -> (131.5, 57.1301) projected
  line L19 (131.5, 57.1301) -> (130.4645, 56.3355) projected
  line L20 (130.4645, 56.3355) -> (129.6699, 55.3) projected
  line L21 (129.6699, 55.3) -> (129.1704, 54.0941) projected
  line L22 (129.1704, 54.0941) -> (129, 52.8) projected
  line L23 (129, 52.8) -> (129.1704, 51.5059) projected
  line L24 (129.1704, 51.5059) -> (129.6699, 50.3) projected
  line L25 (129.6699, 50.3) -> (130.4645, 49.2645) projected
  line L26 (130.4645, 49.2645) -> (131.5, 48.4699) projected
  line L27 (131.5, 48.4699) -> (132.4, 48.0971) projected
  line L28 (132.4, 48.0971) -> (132.4, -5.0172) projected
  arc A16 (131.3636, -6.7698) -> (132.4, -5.0172) centre (130.4, -5.0172) ccw projected
  line L29 (131.3636, -6.7698) -> (128.4686, -8.3615) projected
  arc A17 (127.505, -8.6089) -> (128.4686, -8.3615) centre (127.505, -6.6089) ccw projected
  line L30 (127.505, -8.6089) -> (2.6647, -8.6089) projected
  arc A18 (1.7321, -8.3782) -> (2.6647, -8.6089) centre (2.6647, -6.6089) ccw projected
  line L31 (1.7321, -8.3782) -> (-1.3326, -6.7626) projected
  arc A19 (-2.4, -4.9934) -> (-1.3326, -6.7626) centre (-0.4, -4.9934) ccw projected
  line L32 (-2.4, -4.9934) -> (-2.4, 16.6775) projected
  line L33 (147.8159, -4.2) -> (147.8159, -7.2) projected
  line L34 (147.8159, -7.2) -> (142.8159, -7.2) projected
  line L35 (142.8159, -7.2) -> (142.8159, -4.2) projected
  line L36 (142.8159, -4.2) -> (147.8159, -4.2) projected
  line L37 (-18, 19.2664) -> (-13, 19.2664) projected
  arc A20 (-18, 19.2664) -> (-20, 17.2664) centre (-18, 17.2664) ccw projected
  line L38 (-20, -15.2) -> (-20, 17.2664) projected
  line L39 (-19.9319, -15.7176) -> (-20, -15.2) projected
  line L40 (-19.8478, -15.9654) -> (-19.9319, -15.7176) projected
  line L41 (-19.7321, -16.2) -> (-19.8478, -15.9654) projected
  line L42 (-19.5867, -16.4175) -> (-19.7321, -16.2) projected
  line L43 (-19.4142, -16.6142) -> (-19.5867, -16.4175) projected
  line L44 (-19.2175, -16.7867) -> (-19.4142, -16.6142) projected
  line L45 (-19, -16.9321) -> (-19.2175, -16.7867) projected
  line L46 (-18.7654, -17.0478) -> (-19, -16.9321) projected
  line L47 (-18.5176, -17.1319) -> (-18.7654, -17.0478) projected
  line L48 (-18, -17.2) -> (-18.5176, -17.1319) projected
  line L49 (148, -17.2) -> (-18, -17.2) projected
  line L50 (148.5176, -17.1319) -> (148, -17.2) projected
  line L51 (148.7654, -17.0478) -> (148.5176, -17.1319) projected
  line L52 (149, -16.9321) -> (148.7654, -17.0478) projected
  line L53 (149.2175, -16.7867) -> (149, -16.9321) projected
  line L54 (149.4142, -16.6142) -> (149.2175, -16.7867) projected
  line L55 (149.5867, -16.4175) -> (149.4142, -16.6142) projected
  line L56 (149.7321, -16.2) -> (149.5867, -16.4175) projected
  line L57 (149.8478, -15.9654) -> (149.7321, -16.2) projected
  line L58 (149.9319, -15.7176) -> (149.8478, -15.9654) projected
  line L59 (150, -15.2) -> (149.9319, -15.7176) projected
  line L60 (150, 86.8) -> (150, -15.2) projected
  line L61 (149.9319, 87.3176) -> (150, 86.8) projected
  line L62 (149.8478, 87.5654) -> (149.9319, 87.3176) projected
  line L63 (149.7321, 87.8) -> (149.8478, 87.5654) projected
  line L64 (149.5867, 88.0175) -> (149.7321, 87.8) projected
  line L65 (149.4142, 88.2142) -> (149.5867, 88.0175) projected
  line L66 (149.2175, 88.3867) -> (149.4142, 88.2142) projected
  line L67 (149, 88.5321) -> (149.2175, 88.3867) projected
  line L68 (148.7654, 88.6478) -> (149, 88.5321) projected
  line L69 (148.5176, 88.7319) -> (148.7654, 88.6478) projected
  line L70 (148, 88.8) -> (148.5176, 88.7319) projected
  line L71 (-9, 88.8) -> (148, 88.8) projected
  arc A21 (-9, 88.8) -> (-11, 86.8) centre (-9, 86.8) ccw projected
  line L72 (-11, 21.2664) -> (-11, 86.8) projected
  arc A22 (-13, 19.2664) -> (-11, 21.2664) centre (-13, 21.2664) ccw projected
  line L73 (188.316, 106.5358) -> (-79.5541, 106.5358)
  line L74 (-79.5541, 106.5358) -> (-79.5541, 69.2714)
  line L75 (-79.5541, 69.2714) -> (188.316, 69.2714)
  line L76 (188.316, 69.2714) -> (188.316, 106.5358)
  point P0 (0, 0)
  constraints: 8 end point, 2 parallel, 1 horizontal, 1 perpendicular
extrude "Extrusion5" cut sketch "Sketch7" against normal through all contours L75 L74 L73 L76 L60 L61 L62 L63 L64 L65 L66 L67 L68 L69 L70 L71 A21 L72 | L72 A21 L71 L70 L69 L68 L67 L66 L65 L64 L63 L62 L61 L60 L75
fillet "Fillet8" radius 4 2 edges at (-150, 69.2714, 3) (11, 69.2714, 3)
sketch "Sketch9" plane through (0, 0, 6) normal (0, 0, 1) x (1, 0, 0)
  point P0 (0, 0)
sketch "Sketch10" plane through (0, 0, 0) normal (0, 0, -1) x (-1, 0, 0)
  line L0 (148.479, -2.995) -> (141.36, -2.995)
  line L1 (141.36, -2.995) -> (141.36, -7.2)
  line L2 (141.36, -7.2) -> (148.479, -7.2)
  line L3 (148.479, -7.2) -> (148.479, -2.995)
  point P0 (0, 0)
  constraints: 8 end point, 2 parallel, 1 horizontal, 1 perpendicular
extrude "Extrusion6" add sketch "Sketch10" against normal blind 6
sketch "Sketch11" plane through (0, 0, 0) normal (0, 0, -1) x (-1, 0, 0)
  line L0 (139.8127, 68.2551) -> (139.8127, -15.4379) projected
  line L1 (-18, 19.2664) -> (-13, 19.2664) projected
  line L2 (139.8127, 72.5884) -> (165.3893, 72.5884)
  line L3 (165.3893, 72.5884) -> (165.3893, 19.2664)
  line L4 (165.3893, 19.2664) -> (139.8127, 19.2664)
  line L5 (139.8127, 19.2664) -> (139.8127, 72.5884)
  point P0 (0, 0)
  constraints: 8 end point, 2 parallel, 1 horizontal, 1 perpendicular
extrude "Extrusion7" cut sketch "Sketch11" against normal blind 6
fillet "Fillet9" radius 2 2 edges at (-150, 19.2664, 3) (-139.8127, 19.2664, 3)
body "Solid1"
